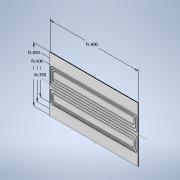
# Autodesk Inventor part: primary_coil_0R2
Saved by Autodesk Inventor 2021 (Build 250183000, 183)
## iProperties
Created: 2021-01-20
Part Number: primary_coil_0R2
Material: Generic
Document SubType Name: Modeling
Designer: phamv
Density: 1 g/cm^3
Appearance: Smooth - White
Author: phamv
Autodesk Inventor part; units mm, degrees
ref_plane "YZ Plane" through (0, 0, 0) normal (1, 0, 0) x (0, 1, 0)
ref_plane "XZ Plane" through (0, 0, 0) normal (0, 1, 0) x (-1, 0, 0)
ref_plane "XY Plane" through (0, 0, 0) normal (0, 0, 1) x (1, 0, 0)
sketch "layer_layout_sketch" plane through (0, 0, 0) normal (0, 0, 1) x (1, 0, 0)
  line L0 (-400, 250) -> (400, 250)
  line L1 (400, 250) -> (400, -250)
  line L2 (400, -250) -> (-400, -250)
  line L3 (-400, -250) -> (-400, 250)
  line L4 (0, 250) -> (0, -250) construction
  line L5 (-400, 200) -> (400, 200)
  line L6 (400, 200) -> (400, -200)
  line L7 (400, -200) -> (-400, -200)
  line L8 (-400, -200) -> (-400, 200)
  line L9 (0, 200) -> (0, -200) construction
  line L10 (-400, 150) -> (400, 150)
  line L11 (400, 150) -> (400, -150)
  line L12 (400, -150) -> (-400, -150)
  line L13 (-400, -150) -> (-400, 150)
  line L14 (0, 150) -> (0, -150) construction
  point P0 (0, 0)
  point P1 (0, 0)
  dimension "d116" = 500
  dimension "d117" = 800
  dimension "d122" = 400
  dimension "d123" = 300
  constraints: 30 end point, 9 midpoint, 6 parallel, 3 horizontal, 3 perpendicular, 2 collinear, 1 coincident, 1 vertical
  measures "d116" distance between parallel lines of L2 L0
  measures "d117" distance between parallel lines of L1 L3
  measures "d122" distance between parallel lines of L7 L5
  measures "d123" distance between parallel lines of L12 L10
sketch "coil_layer_sketch_lower" plane through (0, 0, 0) normal (0, 0, 1) x (1, 0, 0)
  line L0 (0, -9.3) -> (376.5, -9.3)
  line L1 (395, -27.8) -> (395, -131.5)
  line L2 (376.5, -150) -> (-376.5, -150)
  line L3 (-395, -131.5) -> (-395, -50.9)
  line L4 (0, -9.3) -> (0, -13.8)
  line L5 (0, -13.8) -> (375.5, -13.8)
  line L6 (390.5, -28.8) -> (390.5, -130.5)
  line L7 (375.5, -145.5) -> (-375.5, -145.5)
  line L8 (-376.5, -32.4) -> (363.75, -32.4)
  line L9 (382.25, -50.9) -> (382.25, -118.75)
  line L10 (363.75, -137.25) -> (-363.75, -137.25)
  line L11 (-390.5, -130.5) -> (-390.5, -51.9)
  line L12 (-375.5, -36.9) -> (362.75, -36.9)
  line L13 (377.75, -51.9) -> (377.75, -117.75)
  line L14 (362.75, -132.75) -> (-362.75, -132.75)
  line L15 (-377.75, -117.75) -> (-377.75, -75)
  line L16 (-382.25, -118.75) -> (-382.25, -74)
  line L17 (-363.75, -55.5) -> (351, -55.5)
  line L18 (369.5, -74) -> (369.5, -106)
  line L19 (-362.75, -60) -> (350, -60)
  line L20 (365, -75) -> (365, -105)
  line L21 (-558.3641, 0) -> (558.3641, 0) projected
  line L22 (350, -120) -> (-350, -120)
  line L23 (351, -124.5) -> (-351, -124.5)
  line L24 (-369.5, -106) -> (-369.5, -71.7563)
  line L25 (-369.5, -71.7563) -> (-365, -71.7563)
  line L26 (-365, -71.7563) -> (-365, -105)
  arc A0 (395, -27.8) -> (376.5, -9.3) centre (376.5, -27.8) ccw
  arc A1 (382.25, -50.9) -> (363.75, -32.4) centre (363.75, -50.9) ccw
  arc A2 (369.5, -74) -> (351, -55.5) centre (351, -74) ccw
  arc A3 (351, -124.5) -> (369.5, -106) centre (351, -106) ccw
  arc A4 (363.75, -137.25) -> (382.25, -118.75) centre (363.75, -118.75) ccw
  arc A5 (376.5, -150) -> (395, -131.5) centre (376.5, -131.5) ccw
  arc A6 (-395, -131.5) -> (-376.5, -150) centre (-376.5, -131.5) ccw
  arc A7 (-382.25, -118.75) -> (-363.75, -137.25) centre (-363.75, -118.75) ccw
  arc A8 (-369.5, -106) -> (-351, -124.5) centre (-351, -106) ccw
  arc A9 (-376.5, -32.4) -> (-395, -50.9) centre (-376.5, -50.9) ccw
  arc A10 (-363.75, -55.5) -> (-382.25, -74) centre (-363.75, -74) ccw
  arc A11 (-375.5, -36.9) -> (-390.5, -51.9) centre (-375.5, -51.9) ccw
  arc A12 (-362.75, -60) -> (-377.75, -75) centre (-362.75, -75) ccw
  arc A13 (-390.5, -130.5) -> (-375.5, -145.5) centre (-375.5, -130.5) ccw
  arc A14 (-377.75, -117.75) -> (-362.75, -132.75) centre (-362.75, -117.75) ccw
  arc A15 (-365, -105) -> (-350, -120) centre (-350, -105) ccw
  arc A16 (350, -120) -> (365, -105) centre (350, -105) ccw
  arc A17 (362.75, -132.75) -> (377.75, -117.75) centre (362.75, -117.75) ccw
  arc A18 (375.5, -145.5) -> (390.5, -130.5) centre (375.5, -130.5) ccw
  arc A19 (377.75, -51.9) -> (362.75, -36.9) centre (362.75, -51.9) ccw
  arc A20 (390.5, -28.8) -> (375.5, -13.8) centre (375.5, -28.8) ccw
  arc A21 (365, -75) -> (350, -60) centre (350, -75) ccw
  point P0 (0, 0)
  point P1 (0, 0)
  point P2 (368.0934, -60)
  point P3 (370, -61.9066)
  point P4 (0, -150)
  dimension "d1" = 4.5
  dimension "d2" = 4.5
  dimension "d3" = 4.5
  dimension "d4" = 9.3
  dimension "d5" = 790
  dimension "d6" = 395
  dimension "d7" = 4.5
  dimension "d8" = 4.5
  dimension "d9" = 8.25
  dimension "d10" = 4.5
  dimension "d11" = 18.6
  dimension "d12" = 4.5
  dimension "d13" = 8.25
  dimension "d14" = 4.5
  dimension "d15" = 4.5
  dimension "d16" = 4.5
  dimension "d17" = 8.25
  dimension "d19" = 18.6
  dimension "d20" = 8.25
  dimension "d82" = 150
  dimension "d88" = 4.5
  dimension "d89" = 8.25
  dimension "d96" = 4.5
  dimension "d97" = 8.25
  dimension "d98" = 18.5
  dimension "d99" = 15
  dimension "d109" = 15
  constraints: 52 end point, 44 point on circle, 44 tangent, 22 centre point, 19 equal radius, 15 perpendicular, 4 horizontal, 4 vertical, 3 parallel, 1 coincident, 1 midpoint
  measures "d1" distance between parallel lines of L5 L0
  measures "d2" distance between parallel lines of L6 L1
  measures "d3" distance between parallel lines of L2 L7
  measures "d4" distance from line of L21 L0.start
  measures "d5" distance between parallel lines of L3 L1
  measures "d6" distance from line of point (0, 0) L1
  measures "d7" distance between parallel lines of L3 L11
  measures "d8" distance between parallel lines of L13 L9
  measures "d9" distance between parallel lines of L9 L6
  measures "d10" distance between parallel lines of L8 L12
  measures "d11" distance between parallel lines of L8 L5
  measures "d12" distance between parallel lines of L10 L14
  measures "d13" distance between parallel lines of L7 L10
  measures "d14" distance between parallel lines of L16 L15
  measures "d15" distance between parallel lines of L17 L19
  measures "d16" distance between parallel lines of L20 L18
  measures "d17" distance between parallel lines of L18 L13
  measures "d19" distance between parallel lines of L17 L12
  measures "d20" distance between parallel lines of L11 L16
  measures "d82" distance between parallel lines of L2 L21
  measures "d88" distance between parallel lines of L23 L22
  measures "d89" distance between parallel lines of L14 L23
  measures "d96" distance between parallel lines of L24 L26
  measures "d97" distance between parallel lines of L15 L24
  measures "d98" radius of A0
  measures "d99" radius of A11
  measures "d109" radius of A21
sketch "coil_layer_sketch_upper" plane through (0, 0, 0) normal (0, 0, 1) x (1, 0, 0)
  line L0 (0, -13.8) -> (-376.5, -13.8)
  line L1 (-395, 4.7) -> (-395, 131.5)
  line L2 (-376.5, 150) -> (376.5, 150)
  line L3 (395, 131.5) -> (395, 27.8)
  line L4 (0, -9.3) -> (-375.5, -9.3)
  line L5 (-390.5, 5.7) -> (-390.5, 130.5)
  line L6 (-375.5, 145.5) -> (375.5, 145.5)
  line L7 (390.5, 130.5) -> (390.5, 28.8)
  line L8 (375.5, 13.8) -> (-362.75, 13.8)
  line L9 (-377.75, 28.8) -> (-377.75, 117.75)
  line L10 (376.5, 9.3) -> (-363.75, 9.3)
  line L11 (-382.25, 27.8) -> (-382.25, 118.75)
  line L12 (-362.75, 132.75) -> (362.75, 132.75)
  line L13 (-363.75, 137.25) -> (363.75, 137.25)
  line L14 (377.75, 117.75) -> (377.75, 51.9)
  line L15 (362.75, 36.9) -> (-350, 36.9)
  line L16 (382.25, 118.75) -> (382.25, 50.9)
  line L17 (363.75, 32.4) -> (-351, 32.4)
  line L18 (-365, 51.9) -> (-365, 105)
  line L19 (-350, 120) -> (350, 120)
  line L20 (365, 105) -> (365, 75)
  line L21 (350, 60) -> (-356.75, 60)
  line L22 (-369.5, 50.9) -> (-369.5, 106)
  line L23 (-351, 124.5) -> (351, 124.5)
  line L24 (369.5, 106) -> (369.5, 74)
  line L25 (351, 55.5) -> (-356.75, 55.5)
  line L26 (-356.75, 60) -> (-356.75, 55.5)
  line L27 (-700, 0) -> (700, 0)
  line L28 (-980, 0) -> (980, 0) projected
  line L29 (0, -13.8) -> (0, -9.3)
  line L30 (0, -51.9241) -> (0, 188.1241) projected
  arc A0 (365, 105) -> (350, 120) centre (350, 105) ccw
  arc A1 (350, 60) -> (365, 75) centre (350, 75) ccw
  arc A2 (377.75, 117.75) -> (362.75, 132.75) centre (362.75, 117.75) ccw
  arc A3 (362.75, 36.9) -> (377.75, 51.9) centre (362.75, 51.9) ccw
  arc A4 (390.5, 130.5) -> (375.5, 145.5) centre (375.5, 130.5) ccw
  arc A5 (375.5, 13.8) -> (390.5, 28.8) centre (375.5, 28.8) ccw
  arc A6 (-350, 120) -> (-365, 105) centre (-350, 105) ccw
  arc A7 (-365, 51.9) -> (-350, 36.9) centre (-350, 51.9) ccw
  arc A8 (-377.75, 28.8) -> (-362.75, 13.8) centre (-362.75, 28.8) ccw
  arc A9 (-390.5, 5.7) -> (-375.5, -9.3) centre (-375.5, 5.7) ccw
  arc A10 (-362.75, 132.75) -> (-377.75, 117.75) centre (-362.75, 117.75) ccw
  arc A11 (-375.5, 145.5) -> (-390.5, 130.5) centre (-375.5, 130.5) ccw
  arc A12 (-376.5, 150) -> (-395, 131.5) centre (-376.5, 131.5) ccw
  arc A13 (-363.75, 137.25) -> (-382.25, 118.75) centre (-363.75, 118.75) ccw
  arc A14 (-351, 124.5) -> (-369.5, 106) centre (-351, 106) ccw
  arc A15 (-369.5, 50.9) -> (-351, 32.4) centre (-351, 50.9) ccw
  arc A16 (-382.25, 27.8) -> (-363.75, 9.3) centre (-363.75, 27.8) ccw
  arc A17 (-395, 4.7) -> (-376.5, -13.8) centre (-376.5, 4.7) ccw
  arc A18 (351, 55.5) -> (369.5, 74) centre (351, 74) ccw
  arc A19 (363.75, 32.4) -> (382.25, 50.9) centre (363.75, 50.9) ccw
  arc A20 (376.5, 9.3) -> (395, 27.8) centre (376.5, 27.8) ccw
  arc A21 (395, 131.5) -> (376.5, 150) centre (376.5, 131.5) ccw
  arc A22 (382.25, 118.75) -> (363.75, 137.25) centre (363.75, 118.75) ccw
  arc A23 (369.5, 106) -> (351, 124.5) centre (351, 106) ccw
  point P0 (0, 0)
  point P1 (395, 9.3)
  point P2 (-382.25, 9.3)
  point P3 (0, 150)
  point P4 (-700, 0)
  point P5 (700, 0)
  point P6 (0, 150)
  dimension "d58" = 4.5
  dimension "d59" = 4.5
  dimension "d60" = 4.5
  dimension "d61" = 8.25
  dimension "d62" = 8.25
  dimension "d64" = 4.5
  dimension "d65" = 4.5
  dimension "d66" = 4.5
  dimension "d67" = 8.25
  dimension "d69" = 18.6
  dimension "d70" = 4.5
  dimension "d71" = 4.5
  dimension "d72" = 18.6
  dimension "d73" = 8.25
  dimension "d74" = 8.25
  dimension "d75" = 4.5
  dimension "d77" = 18.6
  dimension "d78" = 4.5
  dimension "d79" = 4.5
  dimension "d80" = 4.5
  dimension "d83" = 150
  dimension "d87" = 8.25
  dimension "d91" = 4.5
  dimension "d92" = 9.3
  dimension "d93" = 790
  dimension "d100" = 15
  dimension "d101" = 18.5
  dimension "d102" = 8.25
  constraints: 56 end point, 48 point on circle, 48 tangent, 24 centre point, 22 equal radius, 16 perpendicular, 5 point on line, 4 horizontal, 4 parallel, 3 vertical, 1 coincident, 1 collinear, 1 midpoint, 3 other
  measures "d58" distance between parallel lines of L1 L5
  measures "d59" distance between parallel lines of L2 L6
  measures "d60" distance between parallel lines of L7 L3
  measures "d61" distance between parallel lines of L13 L6
  measures "d62" distance between parallel lines of L5 L11
  measures "d64" distance between parallel lines of L10 L8
  measures "d65" distance between parallel lines of L14 L16
  measures "d66" distance between parallel lines of L13 L12
  measures "d67" distance between parallel lines of L16 L7
  measures "d69" distance between parallel lines of L4 L10
  measures "d70" distance between parallel lines of L11 L9
  measures "d71" distance between parallel lines of L17 L15
  measures "d72" distance between parallel lines of L8 L17
  measures "d73" distance between parallel lines of L12 L23
  measures "d74" distance between parallel lines of L9 L22
  measures "d75" distance between parallel lines of L23 L19
  measures "d77" distance between parallel lines of L15 L25
  measures "d78" distance between parallel lines of L24 L20
  measures "d79" distance between parallel lines of L25 L21
  measures "d80" distance between parallel lines of L22 L18
  measures "d83" distance of the line from the sketch origin of L2
  measures "d87" distance between parallel lines of L18 L26
  measures "d91" distance between parallel lines of L0 L4
  measures "d92" distance between parallel lines of L28 L4
  measures "d93" distance between parallel lines of L3 L1
  measures "d100" radius of A0
  measures "d101" radius of A12
  measures "d102" distance between parallel lines of L14 L24
extrude "layer_sheet Extrude" add sketch "layer_layout_sketch" along normal blind 4.5
extrude "wire_holes_upper Cut" cut sketch "coil_layer_sketch_upper" along normal blind 4.5 contours L0 A17 L27 A9 L4 L29 | A17 L1 A12 L2 L30 L6 A11 L5 A9 L27 | L30 L8 A5 L7 A4 L6 L2 A21 L3 A20 L10 | L10 A16 L11 A13 L13 L30 L12 A10 L9 A8 L8 | L30 L15 A3 L14 A2 L12 L13 A22 L16 A19 L17 | L17 A15 L22 A14 L23 L30 L19 A6 L18 A7 L15 | L30 L21 A1 L20 A0 L19 L23 A23 L24 A18 L25 | L25 L26 L21 L30
extrude "wire_holes_lower Cut" cut sketch "coil_layer_sketch_lower" along normal blind 4.5
equation "\"d1\" = wire_diameter"
equation "\"d2\" = wire_diameter"
equation "\"d3\" = wire_diameter"
equation "\"d4\" = 0.5 * distance_between_wires"
equation "\"d6\" = 0.5 * track_length"
equation "\"d7\" = wire_diameter"
equation "\"d8\" = wire_diameter"
equation "\"d9\" = distance_between_wires_edge"
equation "\"d10\" = wire_diameter"
equation "\"d11\" = distance_between_wires"
equation "\"d12\" = wire_diameter"
equation "\"d13\" = distance_between_wires_edge"
equation "\"d14\" = wire_diameter"
equation "\"d15\" = wire_diameter"
equation "\"d16\" = wire_diameter"
equation "\"d17\" = distance_between_wires_edge"
equation "\"d19\" = distance_between_wires"
equation "\"d20\" = distance_between_wires_edge"
equation "\"d82\" = 0.5 * track_width"
equation "\"d58\" = wire_diameter"
equation "\"d59\" = wire_diameter"
equation "\"d60\" = wire_diameter"
equation "\"d61\" = distance_between_wires_edge"
equation "\"d62\" = distance_between_wires_edge"
equation "\"d64\" = wire_diameter"
equation "\"d65\" = wire_diameter"
equation "\"d66\" = wire_diameter"
equation "\"d67\" = distance_between_wires_edge"
equation "\"d69\" = distance_between_wires"
equation "\"d70\" = wire_diameter"
equation "\"d71\" = wire_diameter"
equation "\"d72\" = distance_between_wires"
equation "\"d73\" = distance_between_wires_edge"
equation "\"d74\" = distance_between_wires_edge"
equation "\"d75\" = wire_diameter"
equation "\"d77\" = distance_between_wires"
equation "\"d78\" = wire_diameter"
equation "\"d79\" = wire_diameter"
equation "\"d80\" = wire_diameter"
equation "\"d83\" = 0.5 * track_width"
equation "\"wire_diameter\" = 4.5"
equation "\"distance_between_wires\" = -1.2 * wire_diameter + 0.2 * parameter_6"
equation "\"distance_between_wires_edge\" = 8.25"
equation "\"bend_radius_inner\" = 15"
equation "\"bend_radius_outer\" = 18.5"
equation "\"track_width\" = 300"
equation "\"parameter_6\" = 120"
equation "\"track_length\" = 790"
body "Solid6"
